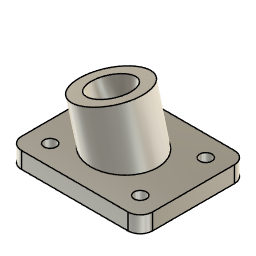
37 (Autodesk Fusion 360 design; units mm, degrees)
Autodesk Fusion 360 part; units mm, degrees
sketch "草图1" plane through (0, 0, 0) normal (0, 0, 1) x (1, 0, 0)
  line L0 (-13, -13) -> (13, -13)
  line L1 (16, -10) -> (16, 10)
  line L2 (13, 13) -> (-13, 13)
  line L3 (-16, 10) -> (-16, -10)
  line L4 (-16, -13) -> (16, 13) construction
  line L5 (16, -13) -> (-16, 13) construction
  circle A0 centre (-11, 8) radius 1.5
  circle A1 centre (-11, -8) radius 1.5
  circle A2 centre (11, 8) radius 1.5
  circle A3 centre (11, -8) radius 1.5
  line L6 (0, 100) -> (0, -100) construction
  line L7 (150, 0) -> (-150, 0) construction
  arc A4 (-13, 13) -> (-16, 10) centre (-13, 10) ccw
  arc A5 (-16, -10) -> (-13, -13) centre (-13, -10) ccw
  arc A6 (13, -13) -> (16, -10) centre (13, -10) ccw
  arc A7 (16, 10) -> (13, 13) centre (13, 10) ccw
  dimension "d1" = 26
  dimension "d2" = 32
  dimension "d3" = 3
  dimension "d4" = 22
  dimension "d5" = 16
  dimension "d6" = 3
  constraint horizontal L0
  constraint perpendicular L0 L1
  constraint parallel L0 L2
  constraint parallel L1 L3
  constraint coincident L4 origin
  constraint coincident L5 origin
  constraint vertical L6
  constraint parallel L2 L7
  constraint symmetric A0.centre A2.centre L6
  constraint symmetric A1.centre A3.centre L6
  constraint symmetric A2.centre A3.centre L7
  constraint equal A2 A3
  constraint equal A0 A1
  constraint equal A0 A2
  constraint coincident L5.end L2
  constraint coincident L5.end L3
  constraint tangent L2 A4
  constraint tangent L3 A4
  constraint coincident L4.start L0
  constraint coincident L4.start L3
  constraint tangent L0 A5
  constraint tangent L3 A5
  constraint equal A4 A5
  constraint coincident L5.start L1
  constraint coincident L5.start L0
  constraint tangent L1 A6
  constraint tangent L0 A6
  constraint equal A4 A6
  constraint coincident L4.end L1
  constraint coincident L4.end L2
  constraint tangent L1 A7
  constraint tangent L2 A7
  constraint equal A4 A7
  measures "d1" distance of L5.start L4.end
  measures "d2" distance of L4.start L5.start
  measures "d3" diameter of A2
  measures "d4" distance of A0.centre A2.centre
  measures "d5" distance of A2.centre A3.centre
  measures "d6" radius of A4
extrude "拉伸1" add sketch "草图1" against normal blind 4 contours L0 L1 L2 L3 A4 A5 A6 A7 picked at (3.253547, -2.385007)
sketch "草图2" plane through (0, 0, 0) normal (0, 1, 0) x (1, 0, 0)
  line L0 (-46.891049, 0) -> (16, 0)
  line L1 (16, 0) -> (16, -16.851606)
  line L2 (16, -16.851606) -> (-46.891049, 0)
  line L3 (-46.891049, 0) -> (-46.891049, 4)
  line L4 (-46.891049, 4) -> (0, 4)
  line L5 (0, 4) -> (16, 4)
  line L6 (16, 0) -> (16, 4)
  line L7 (0, 4) -> (-4.141105, -11.454813) construction
  line L8 (-5.744787, -5.848727) -> (0.050768, -7.401641)
  arc A0 (0.688524, -12.748908) -> (0.050768, -7.401641) centre (-17.302578, -12.183001) ccw
  arc A1 (-5.744787, -5.848727) -> (-8.970734, -10.160718) centre (6.892971, -18.666179) ccw
  line L9 (-4.141105, -11.454813) -> (-2.847009, -6.625184)
  point P0 (-8.970734, -10.160718)
  point P1 (0.688524, -12.748908)
  dimension "d9" = 15
  dimension "d10" = 16
  dimension "d19" = 10
  dimension "d20" = 6
  dimension "d21" = 18
  dimension "d22" = 5
  constraint horizontal L0
  constraint perpendicular L0 L1
  constraint perpendicular L0 L3
  constraint perpendicular L3 L4
  constraint perpendicular L3 L5
  constraint perpendicular L5 L6
  constraint perpendicular L2 L7
  constraint perpendicular L7 L8
  measures "d9" angle of L0 L2
  measures "d10" distance of L2 L4.end
  measures "d21" radius of A0
  measures "d22" distance of L2 L8
sketch "草图3" plane through (0, -13, 0) normal (0, -1, 0) x (1, 0, 0)
  line L0 (13, 0) -> (-13, 0)
  line L1 (-13, 0) -> (-13, -4)
  line L2 (-13, -4) -> (13, -4)
  line L3 (13, -4) -> (13, 0)
  line L4 (16, 16.851606) -> (-46.891049, 0)
ref_plane "工作平面1" through (16, 0, 16.851606) normal (0.258819, 0, -0.965926) x (0, 1, 0)
sketch "草图4" plane through (-3.141105, 0, 11.722762) normal (0.258819, 0, -0.965926) x (0, 1, 0)
  circle A0 centre (0, -1.035276) radius 3
  circle A1 centre (0, -1.035276) radius 5
  circle A2 centre (0, -1.035276) radius 8
  point P0 (0, -1.035276)
  dimension "d11" = 16
  dimension "d12" = 10
  dimension "d13" = 6
  constraint concentric A0 A1
  constraint concentric A0 A2
  measures "d11" diameter of A2
  measures "d12" diameter of A1
  measures "d13" diameter of A0
extrude "拉伸2" add sketch "草图4" along normal up to surface contours A0 | A1 | A2 picked at (-0.755779, -1.072087) picked at (4.303549, -1.432722) picked at (6.9516, -1.681126) end surface through (0, 0, 0) normal (0, 0, 1) offset 0
extrude "拉伸3" cut sketch "草图4" along normal up to surface contours A0 picked at (-0.755779, -1.072087) end surface through (0, 0, -4) normal (0, 0, -1) offset 0
revolve "旋转1" cut sketch "草图2" angle 360 about axis through (0, 0, -4) along (-0.25881905, 0, 0.96592583) contours L2 L8 A1 L9 picked at (-4.650178, -8.418609)
ref_plane "工作平面2" through (20.141105, 0, 1.396793) normal (0.258819, 0, -0.965926) x (0, 1, 0)
sketch "草图5" plane through (1, 0, -3.732051) normal (0.258819, 0, -0.965926) x (0, 1, 0)
  circle A0 centre (0, -1.035276) radius 5
  point P0 (0, -1.035276)
  dimension "d25" = 10
  measures "d25" diameter of A0
extrude "拉伸4" cut sketch "草图5" along normal mid plane 6 contours A0 picked at (0.9146, -2.122601)
